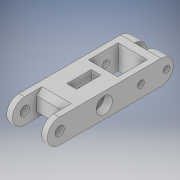
# Autodesk Inventor part: КВ33.044.602 - Держатель катка
Saved by Autodesk Inventor 2019 (Build 230136000, 136)
## iProperties
Created: 2019-07-22
Part Number: КВ33.044.602 - Держатель катка
Material: Типовые
Document SubType Name: Modeling
Designer: user
Density: 1 g/cm^3
Appearance: По умолчанию
Author: user
Autodesk Inventor part; units mm, degrees
ref_plane "YZ Plane" through (0, 0, 0) normal (1, 0, 0) x (0, 1, 0)
ref_plane "XZ Plane" through (0, 0, 0) normal (0, 1, 0) x (-1, 0, 0)
ref_plane "XY Plane" through (0, 0, 0) normal (0, 0, 1) x (1, 0, 0)
sketch "Эскиз1" plane through (0, 0, 0) normal (1, 0, 0) x (0, 1, 0)
  line L0 (-7.5, 25) -> (7.5, 25)
  line L1 (7.5, 25) -> (7.5, -25)
  line L2 (7.5, -25) -> (-7.5, -25)
  line L3 (-7.5, -25) -> (-7.5, 25)
  line L4 (-7.5, 25) -> (7.5, -25) construction
  line L5 (7.5, 25) -> (-7.5, -25) construction
  line L6 (0, -25) -> (0, -32.5)
  arc A0 (-7.5, -32.5) -> (7.5, -32.5) centre (0, -32.5) ccw
  line L7 (-7.5, -25) -> (-7.5, -32.5)
  line L8 (7.5, -25) -> (7.5, -32.5)
  circle A1 centre (0, -32.5) radius 2.1
  line L9 (-7.5, -32.5) -> (-7.5, -44.5)
  line L10 (-7.5, -44.5) -> (7.5, -44.5)
  line L11 (7.5, -44.5) -> (7.5, -32.5)
  line L12 (7.5, -32.5) -> (2.1, -32.5)
  line L13 (-2.1, -32.5) -> (-7.5, -32.5)
  line L14 (7.5, -44.5) -> (-7.5, -44.5)
  line L15 (-7.5, -44.5) -> (-7.5, -52.5)
  line L16 (-7.5, -52.5) -> (7.5, -52.5)
  line L17 (7.5, -52.5) -> (7.5, -44.5)
  point P0 (0, 0)
  dimension "d0" = 15
  dimension "d1" = 50
  dimension "d4" = 4.2
  dimension "d31" = 15
  dimension "d32" = 12
  dimension "d34" = 8
  constraints: 36 end point, 7 parallel, 4 horizontal, 4 perpendicular, 4 point on circle, 3 midpoint, 2 centre point, 2 coincident, 1 point on line, 1 tangent, 1 vertical
  measures "d0" distance of L1.end L2.end
  measures "d1" distance of L0.end L1.end
  measures "d4" diameter of A1
  measures "d31" distance of L10.end L9.end
  measures "d32" distance of L9.end L9.start
  measures "d34" distance of L15.end L14.end
extrude "Выдавливание1" add sketch "Эскиз1" along normal blind 25 contours L0 L1 L2 L3 | L2 L6 A1 L13 L7 | L8 L12 A1 L6 L2 | L13 A1 L12 A0 | A0 L11 L10 L9 | L10 L17 L16 L15
sketch "Эскиз2" plane through (0, 7.5, 25) normal (0, 1, 0) x (1, 0, 0)
  line L0 (0, 65) -> (25, 65) projected
  line L1 (3.5, 50) -> (21.5, 50)
  line L2 (21.5, 50) -> (21.5, 65)
  line L3 (21.5, 65) -> (3.5, 65)
  line L4 (3.5, 65) -> (3.5, 50)
  line L5 (0, 57.5) -> (25, 57.5) projected
  line L6 (3.5, 50) -> (21.5, 65) construction
  line L7 (21.5, 50) -> (3.5, 65) construction
  point P0 (0, 25)
  point P1 (12.5, 57.5)
  dimension "d7" = 18
  constraints: 12 end point, 3 midpoint, 2 parallel, 1 horizontal, 1 perpendicular, 1 point on line
  measures "d7" distance of L3.end L2.end
extrude "Выдавливание2" cut sketch "Эскиз2" against normal blind 25
sketch "Эскиз3" plane through (0, 7.5, 25) normal (0, 1, 0) x (1, 0, 0)
  line L0 (21.5, 50) -> (3.5, 50) projected
  line L1 (12.5, 50) -> (12.5, 35)
  line L2 (9.5, 27.5) -> (15.5, 27.5)
  line L3 (15.5, 27.5) -> (15.5, 42.5)
  line L4 (15.5, 42.5) -> (9.5, 42.5)
  line L5 (9.5, 42.5) -> (9.5, 27.5)
  line L6 (9.5, 27.5) -> (15.5, 42.5) construction
  line L7 (15.5, 27.5) -> (9.5, 42.5) construction
  point P0 (0, 25)
  dimension "d10" = 15
  dimension "d11" = 6
  dimension "d12" = 15
  constraints: 14 end point, 3 midpoint, 2 parallel, 1 horizontal, 1 perpendicular, 1 vertical
  measures "d10" distance of L1.start L1.end
  measures "d11" distance of L4.end L3.end
  measures "d12" distance of L3.end L2.end
extrude "Выдавливание3" cut sketch "Эскиз3" against normal blind 25
sketch "Эскиз4" plane through (25, 0, 0) normal (1, 0, 0) x (0, 0, -1)
  line L0 (2.5, 7.5) -> (2.5, -7.5) projected
  line L1 (17.5, 7.5) -> (17.5, -7.5) projected
  line L2 (2.5, 7.5) -> (2.5, -7.5) projected
  line L3 (2.5, 0) -> (17.5, 0)
  circle A0 centre (10, 0) radius 1.8
  point P0 (0, 0)
  dimension "d15" = 3.6
  constraints: 3 midpoint, 2 end point, 1 centre point
  measures "d15" diameter of A0
extrude "Выдавливание4" cut sketch "Эскиз4" against normal blind 25
sketch "Эскиз5" plane through (25, 0, 0) normal (1, 0, 0) x (0, 0, -1)
  circle A0 centre (10, 0) radius 1.8 projected
  circle A1 centre (10, 0) radius 5
  point P0 (0, 0)
  dimension "d18" = 10
  constraints: 1 centre point, 1 coincident
  measures "d18" diameter of A1
extrude "Выдавливание5" cut sketch "Эскиз5" against normal blind 5
fillet "Сопряжение1" radius 7.5 2 edges at (12.5, 7.5, 25) (12.5, -7.5, 25)
sketch "Эскиз6" plane through (25, 0, 0) normal (1, 0, 0) x (0, 0, -1)
  arc A0 (-17.5, 7.5) -> (-17.5, -7.5) centre (-17.5, 0) ccw projected
  circle A1 centre (-17.5, 0) radius 2.85
  point P0 (0, 0)
  dimension "d22" = 5.7
  constraints: 1 centre point, 1 coincident
  measures "d22" diameter of A1
extrude "Выдавливание6" cut sketch "Эскиз6" against normal blind 25
sketch "Эскиз7" plane through (3.5, 7.5, -25) normal (0, 1, 0) x (1, 0, 0)
  line L0 (-3.5, -50) -> (21.5, -50) projected
  line L1 (0, -35) -> (18, -35)
  line L2 (18, -35) -> (18, -50)
  line L3 (18, -50) -> (0, -50)
  line L4 (0, -50) -> (0, -35)
  line L5 (-3.5, -42.5) -> (21.5, -42.5) projected
  line L6 (0, -35) -> (18, -50) construction
  line L7 (18, -35) -> (0, -50) construction
  point P0 (-3.5, -25)
  point P1 (9, -42.5)
  dimension "d25" = 18
  constraints: 12 end point, 3 midpoint, 2 parallel, 1 horizontal, 1 perpendicular, 1 point on line
  measures "d25" distance of L2.end L3.end
extrude "Выдавливание7" cut sketch "Эскиз7" against normal blind 25
chamfer "Фаска1" distance 3.25 angle 45 4 edges at (12.5, 7.5, 10) (12.5, -7.5, 10) (12.5, 7.5, -25) (12.5, -7.5, -25)
fillet "Сопряжение3" radius 7.5 2 edges at (12.5, 7.5, -52.5) (12.5, -7.5, -52.5)
sketch "Эскиз8" plane through (25, 0, 0) normal (1, 0, 0) x (0, 0, -1)
  circle A0 centre (48.2471, 0) radius 2
  point P0 (0, 0)
  dimension "d36" = 4
  constraints: 1 centre point
  measures "d36" diameter of A0
extrude "Выдавливание8" cut sketch "Эскиз8" against normal blind 25
sketch "Эскиз9" plane through (0, 7.5, 17.5) normal (0, 1, 0) x (1, 0, 0)
  line L0 (25, 62.5) -> (0, 62.5) projected
  line L1 (0, 70) -> (25, 70) projected
  line L2 (8.611, 62.5) -> (15.9557, 62.5)
  line L3 (15.9557, 62.5) -> (15.9557, 70)
  line L4 (15.9557, 70) -> (8.611, 70)
  line L5 (8.611, 70) -> (8.611, 62.5)
  point P0 (0, 17.5)
  constraints: 8 end point, 2 parallel, 2 point on line, 1 horizontal, 1 perpendicular
extrude "Выдавливание9" cut sketch "Эскиз9" against normal blind 25
